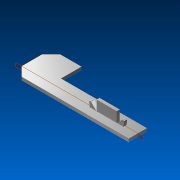
# Autodesk Inventor part: Soanar Power Module Pin E
Saved by Autodesk Inventor 2016 (Build 200138000, 138)
## iProperties
Created: 2013-08-06
Part Number: Soanar Power Module Pin E
Material: Nickel-Copper Alloy 400
Document SubType Name: Modeling
Designer: sdarley
Density: 8.83 g/cm^3
Appearance: Chrome - Polished
Author: sdarley
Autodesk Inventor part; units mm, degrees
ref_plane "YZ Plane" through (0, 0, 0) normal (1, 0, 0) x (0, 1, 0)
ref_plane "XZ Plane" through (0, 0, 0) normal (0, 1, 0) x (-1, 0, 0)
ref_plane "XY Plane" through (0, 0, 0) normal (0, 0, 1) x (1, 0, 0)
sketch "Sketch1" plane through (0, 0, 0) normal (0, 0, 1) x (1, 0, 0)
  line L0 (0, 0) -> (-18, 0)
  line L1 (-18, 0) -> (-19.55, 1.55)
  line L2 (-19.55, 1.55) -> (-19.55, 4.95)
  line L3 (-19.55, 4.95) -> (-18, 6.5)
  line L4 (-18, 6.5) -> (-14.45, 6.5)
  line L5 (-14.45, 6.5) -> (-14.45, 3.05)
  line L6 (-14.45, 3.05) -> (0, 3.05)
  line L7 (0, 3.05) -> (0, 0)
  point P0 (-19.55, 3.25)
  dimension "d0" = 3.05
  dimension "d1" = 14.45
  dimension "d2" = 6.5
  dimension "d3" = 5.1
  dimension "d4" = 3.4
  dimension "d5" = 3.25
  dimension "d6" = 3.55
  constraints: 16 end point, 4 parallel, 1 horizontal, 1 midpoint, 1 perpendicular, 1 vertical alignment
  measures "d0" distance between parallel lines of L0 L6
  measures "d1" distance of L5.end L6.end
  measures "d2" distance between parallel lines of L0 L4
  measures "d3" distance between parallel lines of L2 L5
  measures "d4" distance of L1.end L2.end
  measures "d5" distance from line of L4 point (-19.55, 3.25)
  measures "d6" distance of L3.end L4.end
extrude "Extrusion1" add sketch "Sketch1" along normal blind 0.55
ref_plane "Work Plane1" through (-14.45, 1.525, 0) normal (0, 1, 0) x (1, 0, 0)
sketch "Sketch2" plane through (-14.45, 1.525, 0) normal (0, 1, 0) x (1, 0, 0)
  line L0 (14.45, -0.55) -> (0, -0.55) projected
  line L1 (14.45, 0) -> (14.45, -0.55) projected
  line L2 (7.75, -0.55) -> (11.15, -0.55)
  line L3 (11.15, -0.55) -> (11.15, -2.25)
  line L4 (11.15, -2.25) -> (7.75, -2.25)
  line L5 (7.75, -2.25) -> (7.75, -0.55)
  line L6 (11.15, -0.55) -> (12.475, -1.875)
  line L7 (12.475, -1.875) -> (12.275, -0.55)
  line L8 (7.75, -0.55) -> (6.425, -1.875)
  line L9 (6.425, -1.875) -> (6.625, -0.55)
  line L10 (6.625, -0.55) -> (7.75, -0.55)
  line L11 (11.15, -0.55) -> (12.275, -0.55)
  point P0 (9.45, -2.25)
  dimension "d9" = 3.3
  dimension "d10" = 3.4
  dimension "d11" = 1.7
  dimension "d14" = 6.05
  dimension "d15" = 3.025
  dimension "d16" = 5.65
  constraints: 20 end point, 3 point on line, 2 collinear, 2 equal length, 2 parallel, 2 perpendicular, 1 horizontal, 1 midpoint
  measures "d9" distance between parallel lines of L3 L1
  measures "d10" distance between parallel lines of L5 L3
  measures "d11" distance between parallel lines of L0 L4
  measures "d14" distance of L6.end L8.end
  measures "d15" horizontal distance of point (9.45, -2.25) L8.end
  measures "d16" distance of L7.end L9.end
extrude "Extrusion2" add sketch "Sketch2" along normal mid plane 0.5
fillet "Fillet1" radius 0.2 2 edges at (-8.025, 1.525, 1.875) (-1.975, 1.525, 1.875)
equation "\"d5\" = 0.5 * d2"
equation "\"d15\" = 0.5 * d14"
body "Solid1"
